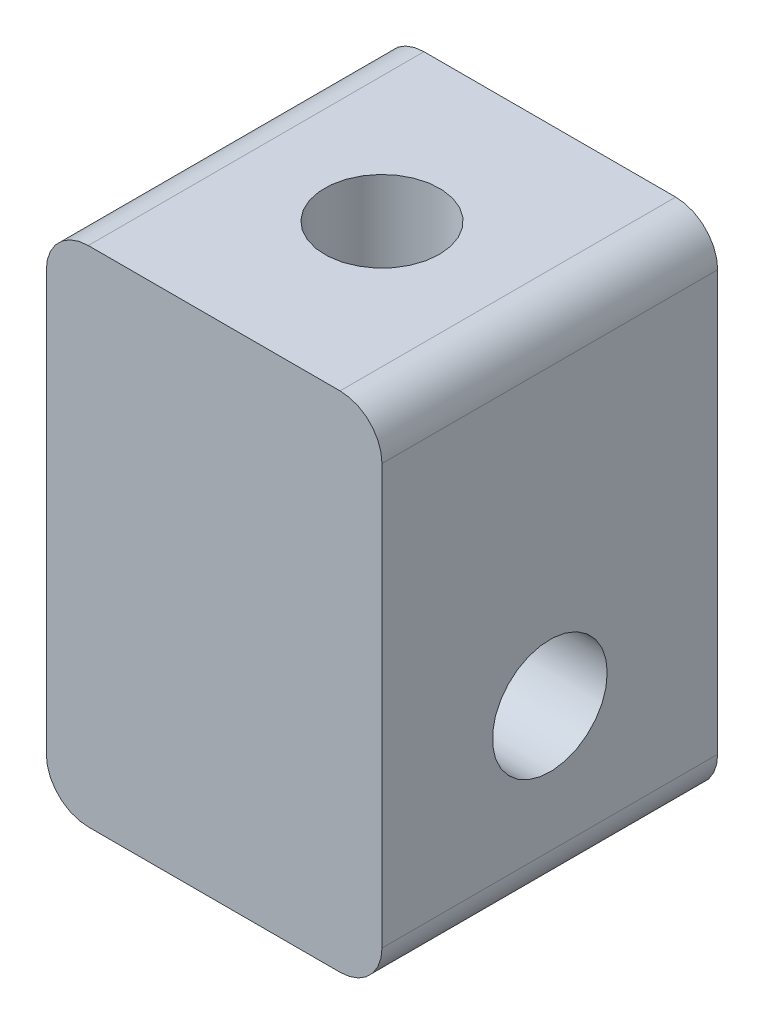
# Autodesk Inventor part: PLATE,NUT-BLOCK,SINGLE-L
Saved by Autodesk Inventor 2026 (Build 300175000, 175)
## iProperties
Created: 2026-02-09
Part Number: PLATE,NUT-BLOCK,SINGLE-L
Material: Aluminum 6061
Document SubType Name: Sheet Metal
Designer: littl
Density: 2.7 g/cm^3
Sheet Metal Rule: Default
Appearance: Aluminum - Flat
Author: littl
Autodesk Inventor part; units mm, degrees
ref_plane "YZ Plane" through (0, 0, 0) normal (1, 0, 0) x (0, 1, 0)
ref_plane "XZ Plane" through (0, 0, 0) normal (0, 1, 0) x (-1, 0, 0)
ref_plane "XY Plane" through (0, 0, 0) normal (0, 0, 1) x (1, 0, 0)
sketch "Sketch1" plane through (0, 0, 0) normal (0, 0, 1) x (1, 0, 0)
  line L0 (6.35, -9.525) -> (-6.35, -9.525)
  line L1 (-6.35, -9.525) -> (-6.35, 9.525)
  line L2 (-6.35, 9.525) -> (6.35, 9.525)
  line L3 (6.35, 9.525) -> (6.35, -9.525)
  line L4 (6.35, -9.525) -> (-6.35, 9.525) construction
  line L5 (-6.35, -9.525) -> (6.35, 9.525) construction
  point P0 (0, 0)
  dimension "d0" = 12.7
  dimension "d1" = 19.05
  measures "d0" distance of L1.end L2.end
  measures "d1" distance of L0.end L1.end
extrude "Plate1" add sketch "Sketch1" along normal blind 12.7
sketch "Sketch2" plane through (-6.35, 9.525, 0) normal (0, 1, 0) x (1, 0, 0)
  line L0 (12.7, 0) -> (0, 0) projected
  point P0 (6.35, 0)
  point P1 (6.35, -6.35)
  point P2 (6.35, 0)
  dimension "d3" = 6.35
  constraints: 1 midpoint, 1 vertical alignment
  measures "d3" distance from line of L0 point (6.35, -6.35)
hole "Hole1" at (0, 9.525, 6.35) direction (0, -1, 0) diameter 4.3434 depth 6.35 tip angle 118 thread size "12-24 UNC" class "2B" standard "ANSI Unified Screw Threads"
sketch "Sketch3" plane through (6.35, -9.525, 0) normal (1, 0, 0) x (0, 0, -1)
  line L0 (0, 19.05) -> (-12.7, 19.05) projected
  point P0 (0, 9.525)
  point P1 (-6.35, 6.35)
  point P2 (-6.35, 19.05)
  dimension "d11" = 12.7
  constraints: 1 midpoint, 1 vertical alignment
  measures "d11" distance from line of L0 point (-6.35, 6.35)
hole "Hole2" at (6.35, -3.175, 6.35) direction (-1, 0, 0) diameter 4.3434 depth 12.7 thread size "12-24 UNC" class "2B" standard "ANSI Unified Screw Threads"
fillet "Corner Round1" radius 1.5875 4 edges at (6.35, 9.525, 6.35) (-6.35, 9.525, 6.35) (-6.35, -9.525, 6.35) (6.35, -9.525, 6.35)
equation "\"d17\" = Thickness"
equation "\"d2\" = Thickness"
equation "\"BendRadius\" = Thickness"
equation "\"BendReliefWidth\" = Thickness"
equation "\"BendReliefDepth\" = 0.5 * Thickness"
equation "\"CornerReliefSize\" = 4 * Thickness"
equation "\"MinimumRemnant\" = 2 * Thickness"
equation "\"TransitionRadius\" = BendRadius"
equation "\"JacobiRadiusSize\" = BendRadius"
equation "\"GapSize\" = Thickness"
equation "\"Thickness\" = 12.7"
body "Solid1"
